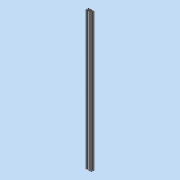
# Autodesk Inventor part: Profil dolny długi
Saved by Autodesk Inventor 2018 (Build 220112000, 112)
## iProperties
Created: 2019-01-21
Part Number: Profil dolny długi
Material: Ogólny
Document SubType Name: Modeling
Designer: Dawid
Density: 1 g/cm^3
Appearance: Aluminium odlewane
Author: Dawid
Autodesk Inventor part; units mm, degrees
ref_plane "YZ Plane" through (0, 0, 0) normal (1, 0, 0) x (0, 1, 0)
ref_plane "XZ Plane" through (0, 0, 0) normal (0, 1, 0) x (-1, 0, 0)
ref_plane "XY Plane" through (0, 0, 0) normal (0, 0, 1) x (1, 0, 0)
sketch "Szkic1" plane through (0, 0, 0) normal (0, 0, 1) x (1, 0, 0)
  circle A0 centre (-10, 9.9979) radius 2.1
  line L0 (-14.9697, 3.9697) -> (-13.0393, 5.9)
  line L1 (-18.0066, 4.5634) -> (-18.0066, 6.2992)
  line L2 (-18.0066, 13.7008) -> (-18.0066, 15.4396)
  line L3 (-14.9697, 3.9697) -> (-15.4393, 3.5)
  line L4 (-13.7036, 2) -> (-15.4393, 2)
  line L5 (-13.5697, 14.6303) -> (-15.4393, 16.5)
  line L6 (-13.5697, 14.6303) -> (-13.0393, 14.1)
  line L7 (-14.641, 13.5721) -> (-14.1103, 13.0421)
  line L8 (-13.7022, 18.0033) -> (-15.4393, 18.0033)
  line L9 (-14.641, 13.5721) -> (-16.5118, 15.4406)
  line L10 (-15.4393, 18.0033) -> (-15.4393, 16.5)
  line L11 (-18.0066, 15.4396) -> (-16.5118, 15.4406)
  line L12 (-18.0066, 4.5634) -> (-16.5066, 4.5634)
  line L13 (-15.4393, 2) -> (-15.4393, 3.5)
  line L14 (-6.4303, 14.6303) -> (-6.9607, 14.1)
  line L15 (-5.3697, 13.5744) -> (-5.9, 13.044)
  line L16 (-5.9, 4.8393) -> (-6.9607, 5.9)
  line L17 (0, 2.0047) -> (-0.9393, 2.0047)
  line L18 (0, 18.0047) -> (-0.9393, 18.0047)
  line L19 (-6.4303, 14.6303) -> (-4.5607, 16.5)
  line L20 (-3.0607, 18.0047) -> (-3.0607, 15.8834)
  line L21 (-3.0607, 18.0047) -> (-0.9393, 18.0047)
  line L22 (-5.3697, 13.5744) -> (-3.0607, 15.8834)
  line L23 (-3.0607, 2.0047) -> (-3.0607, 4.126)
  line L24 (-5.9, 4.8393) -> (-4.5607, 3.5)
  line L25 (-3.0607, 2.0047) -> (-0.9393, 2.0047)
  line L26 (-14.1088, 10.5027) -> (-14.1103, 13.0421)
  line L27 (-10.5, 14.1) -> (-13.0393, 14.1)
  line L28 (-9.5, 14.1) -> (-6.9607, 14.1)
  line L29 (-5.9, 10.5047) -> (-5.9, 13.044)
  line L30 (-5.9, 9.5047) -> (-5.9, 6.9653)
  line L31 (-9.5, 5.9) -> (-6.9607, 5.9)
  line L32 (-10.5, 5.9) -> (-13.0393, 5.9)
  arc A1 (-10.5, 14.1) -> (-9.5, 14.1) centre (-10, 14.6) ccw
  arc A2 (-14.1066, 9.5043) -> (-14.1088, 10.5027) centre (-14.6085, 10.0024) ccw
  arc A3 (-9.5, 5.9) -> (-10.5, 5.9) centre (-10, 5.4) ccw
  arc A4 (-5.9, 10.5047) -> (-5.9, 9.5047) centre (-5.4, 10.0047) ccw
  circle A5 centre (10.0007, 9.9979) radius 2.1
  line L33 (14.9679, 3.971) -> (13.0384, 5.9021)
  line L34 (15.4994, 6.8934) -> (15.1709, 6.8935) construction
  line L35 (18.0049, 4.5557) -> (18.0049, 6.2915)
  line L36 (18.0109, 13.6978) -> (18.0112, 15.4336)
  line L37 (14.9679, 3.971) -> (15.4374, 3.5011)
  line L38 (13.7009, 2.0011) -> (15.4367, 2.0011)
  line L39 (13.5723, 14.6246) -> (15.4428, 16.4934)
  line L40 (13.5723, 14.6246) -> (13.0418, 14.0945)
  line L41 (14.6404, 13.5661) -> (14.1097, 13.0361)
  line L42 (13.7076, 17.9967) -> (15.4434, 17.9967)
  line L43 (14.6404, 13.5661) -> (16.5112, 15.4346)
  line L44 (15.4434, 17.9967) -> (15.4428, 16.4934)
  line L45 (18.0112, 15.4336) -> (16.5112, 15.4346)
  line L46 (18.0049, 4.5557) -> (16.5049, 4.5564)
  line L47 (15.4367, 2.0011) -> (15.4374, 3.5011)
  line L48 (6.433, 14.6276) -> (6.9631, 14.097)
  line L49 (5.3719, 13.5721) -> (5.902, 13.0415)
  line L50 (5.8986, 4.8445) -> (6.9597, 5.9047)
  line L51 (0, 2.0047) -> (0.9366, 2.0043)
  line L52 (0, 18.0047) -> (0.9434, 18.0043)
  line L53 (4.5647, 17.9981) -> (4.5641, 16.4981)
  line L54 (6.433, 14.6276) -> (4.5641, 16.4981)
  line L55 (3.0648, 18.0034) -> (3.0638, 15.8821)
  line L56 (3.0648, 18.0034) -> (0.9434, 18.0043)
  line L57 (5.3719, 13.5721) -> (3.0638, 15.8821)
  line L58 (3.0579, 2.0034) -> (3.0588, 4.1247)
  line L59 (5.8986, 4.8445) -> (4.5587, 3.5057)
  line L60 (3.0579, 2.0034) -> (0.9366, 2.0043)
  line L61 (14.1082, 10.4967) -> (14.1097, 13.0361)
  line L62 (10.5024, 14.0955) -> (13.0418, 14.0945)
  line L63 (9.5024, 14.096) -> (6.9631, 14.097)
  line L64 (5.9009, 10.5022) -> (5.902, 13.0415)
  line L65 (5.9005, 9.5022) -> (5.8994, 6.9628)
  line L66 (9.499, 5.9036) -> (6.9597, 5.9047)
  line L67 (10.499, 5.9032) -> (13.0384, 5.9021)
  arc A6 (9.5024, 14.096) -> (10.5024, 14.0955) centre (10.0026, 14.5957) ccw
  arc A7 (14.1082, 10.4967) -> (14.106, 9.4983) centre (14.6078, 9.9964) ccw
  arc A8 (10.499, 5.9032) -> (9.499, 5.9036) centre (9.9988, 5.4034) ccw
  arc A9 (5.9005, 9.5022) -> (5.9009, 10.5022) centre (5.4007, 10.0024) ccw
  arc A10 (-13.7022, 18.0033) -> (-13.5268, 18.4268) centre (-13.7022, 18.2514) ccw
  arc A11 (-6.4665, 18.4282) -> (-6.2912, 18.0046) centre (-6.2911, 18.2527) ccw
  arc A12 (6.3005, 17.9973) -> (6.4748, 18.4175) centre (6.3006, 18.2435) ccw
  arc A13 (13.5336, 18.4169) -> (13.7076, 17.9967) centre (13.7076, 18.2429) ccw
  arc A14 (18.0109, 13.6978) -> (18.4311, 13.5237) centre (18.257, 13.6978) ccw
  arc A15 (18.4251, 6.4656) -> (18.0049, 6.2915) centre (18.2511, 6.2915) ccw
  arc A16 (13.7009, 2.0011) -> (13.5269, 1.5809) centre (13.7009, 1.7549) ccw
  arc A17 (-6.2915, 2.0047) -> (-6.4671, 1.586) centre (-6.2915, 1.7585) ccw
  arc A18 (-13.5295, 1.5798) -> (-13.7036, 2) centre (-13.7036, 1.7538) ccw
  arc A19 (-18.0066, 6.2992) -> (-18.4268, 6.4732) centre (-18.2527, 6.2992) ccw
  arc A20 (-18.4268, 13.5268) -> (-18.0066, 13.7008) centre (-18.2527, 13.7008) ccw
  line L68 (-4.5607, 16.5) -> (-4.5607, 18.0046)
  line L69 (-6.2912, 18.0046) -> (-4.5607, 18.0046)
  line L70 (6.3005, 17.9973) -> (4.5647, 17.9981)
  line L71 (-14.1066, 9.5043) -> (-14.1066, 6.9634)
  line L72 (14.106, 9.4983) -> (14.106, 6.9574)
  line L73 (3.0588, 4.1247) -> (5.8994, 6.9628)
  line L74 (-5.9, 6.9653) -> (-3.0607, 4.126)
  line L75 (-4.5607, 2.0047) -> (-6.2915, 2.0047)
  line L76 (-4.5607, 3.5) -> (-4.5607, 2.0047)
  line L77 (4.5587, 2.0034) -> (6.3693, 2.0034)
  line L78 (6.5461, 1.5766) -> (6.5038, 1.5343)
  line L79 (4.5587, 3.5057) -> (4.5587, 2.0034)
  arc A21 (6.5461, 1.5766) -> (6.3693, 2.0034) centre (6.3693, 1.7534) ccw
  line L80 (-20, 18.0132) -> (-20, 18.0033)
  line L81 (-18.4268, 13.5268) -> (-19.9268, 15.0268)
  line L82 (-13.5268, 18.4268) -> (-15.0528, 19.9528)
  line L83 (-6.4665, 18.4282) -> (-4.9418, 19.9528)
  line L84 (6.4748, 18.4175) -> (4.9394, 19.9528)
  line L85 (13.5336, 18.4169) -> (15.0694, 19.9528)
  line L86 (18.4311, 13.5237) -> (19.9268, 15.0194)
  line L87 (13.5269, 1.5809) -> (15.0085, 0.0992)
  line L88 (6.5038, 1.5343) -> (5.0687, 0.0992)
  line L89 (-6.4671, 1.586) -> (-4.9803, 0.0992)
  line L90 (-13.5295, 1.5798) -> (-15.0101, 0.0992)
  line L91 (-18.4268, 6.4732) -> (-19.9268, 4.9732)
  line L92 (-15.2296, 20.026) -> (-19.5, 20.026)
  line L93 (19.5, 20.026) -> (15.2462, 20.026)
  line L94 (4.7627, 20.026) -> (-4.7651, 20.026)
  line L95 (20, 0.526) -> (20, 4.7886)
  line L96 (20, 15.1962) -> (20, 19.526)
  line L97 (15.1853, 0.026) -> (19.5, 0.026)
  line L98 (-19.5, 0.026) -> (-15.1868, 0.026)
  line L99 (-4.8035, 0.026) -> (4.8919, 0.026)
  line L100 (-20, 19.526) -> (-20, 15.2036)
  line L101 (-20, 4.7964) -> (-20, 0.526)
  line L102 (-16.5066, 4.5634) -> (-14.1066, 6.9634)
  line L103 (16.5049, 4.5564) -> (14.106, 6.9574)
  line L104 (18.4251, 6.4656) -> (19.9267, 4.9655)
  line L105 (-8.9462, 9.9979) -> (-8.9325, 9.9979)
  arc A22 (-15.0528, 19.9528) -> (-15.2296, 20.026) centre (-15.2296, 19.776) ccw
  arc A23 (-20, 15.2036) -> (-19.9268, 15.0268) centre (-19.75, 15.2036) ccw
  arc A24 (-19.9268, 4.9732) -> (-20, 4.7964) centre (-19.75, 4.7964) ccw
  arc A25 (-15.1868, 0.026) -> (-15.0101, 0.0992) centre (-15.1868, 0.276) ccw
  arc A26 (-4.9803, 0.0992) -> (-4.8035, 0.026) centre (-4.8035, 0.276) ccw
  arc A27 (4.8919, 0.026) -> (5.0687, 0.0992) centre (4.8919, 0.276) ccw
  arc A28 (15.0085, 0.0992) -> (15.1853, 0.026) centre (15.1853, 0.276) ccw
  arc A29 (20, 4.7886) -> (19.9267, 4.9655) centre (19.75, 4.7886) ccw
  arc A30 (19.9268, 15.0194) -> (20, 15.1962) centre (19.75, 15.1962) ccw
  arc A31 (15.2462, 20.026) -> (15.0694, 19.9528) centre (15.2462, 19.776) ccw
  arc A32 (4.9394, 19.9528) -> (4.7627, 20.026) centre (4.7627, 19.776) ccw
  arc A33 (-4.7651, 20.026) -> (-4.9418, 19.9528) centre (-4.7651, 19.776) ccw
  arc A34 (-19.5, 20.026) -> (-20, 19.526) centre (-19.5, 19.526) ccw
  arc A35 (20, 19.526) -> (19.5, 20.026) centre (19.5, 19.526) ccw
  arc A36 (19.5, 0.026) -> (20, 0.526) centre (19.5, 0.526) ccw
  arc A37 (-20, 0.526) -> (-19.5, 0.026) centre (-19.5, 0.526) ccw
  dimension "d103" = 0.25
  dimension "d104" = 0.5
  constraints: 212 end point, 72 point on circle, 42 tangent, 38 centre point, 23 equal radius, 13 parallel, 10 horizontal, 8 perpendicular, 6 point on line, 6 vertical
  measures "d103" radius of A22
  measures "d104" radius of A34
extrude "Wyciągnięcie proste2" add sketch "Szkic1" along normal blind 1000
